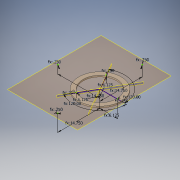
# Autodesk Inventor part: newCam08
Saved by Autodesk Inventor 2016 (Build 200138000, 138)
## iProperties
Created: 2015-07-25
Part Number: newCam08
Material: Generic
Document SubType Name: Modeling
Designer: steele
Density: 1 g/cm^3
Appearance: Default
Author: steele
Autodesk Inventor part; units mm, degrees
ref_plane "YZ Plane" through (0, 0, 0) normal (1, 0, 0) x (0, 1, 0)
ref_plane "XY Plane" through (0, 0, 0) normal (0, 0, 1) x (1, 0, 0)
sketch "Sketch1" plane through (0, 0, 0) normal (0, 1, 0) x (-1, 0, 0)
  circle A0 centre (0, 0) radius 149.225
  circle A1 centre (0, 0) radius 187.325
  dimension "insideCamDiam" = 298.45
  dimension "outsideCamDiam" = 374.65
  constraints: 2 centre point, 1 coincident
  measures "insideCamDiam" diameter of A0
  measures "outsideCamDiam" diameter of A1
extrude "Extrusion1" add sketch "Sketch1" against normal blind 12.7
sketch "Sketch yz neg" plane through (0, 0, 0) normal (1, 0, 0) x (0, 1, 0)
  circle A0 centre (0, -374.65) radius 3.175
  point P0 (0, 0)
  dimension "trackDiam" = 6.35
  dimension "yzNetOutsideCamTrackRadius" = 374.65
  constraints: 1 centre point
  measures "trackDiam" diameter of A0
  measures "yzNetOutsideCamTrackRadius" distance of point (0, 0) A0.centre
sketch "Sketch xy neg" plane through (0, 0, 0) normal (0, 0, 1) x (1, 0, 0)
  circle A0 centre (-374.65, 0) radius 3.175
  point P0 (0, 0)
  dimension "xyNegTrackDiam" = 6.35
  dimension "xyNegOutsideCamTrackRadius" = 374.65
  constraints: 1 centre point
  measures "xyNegTrackDiam" diameter of A0
  measures "xyNegOutsideCamTrackRadius" distance of point (0, 0) A0.centre
sketch "Sketch yz pos" plane through (0, 0, 0) normal (1, 0, 0) x (0, 1, 0)
  circle A0 centre (0, 374.65) radius 3.175
  point P0 (0, 0)
  dimension "yzOutsideCamTrackRadius" = 374.65
  dimension "yzPosTrackDiam" = 6.35
  constraints: 1 centre point
  measures "yzOutsideCamTrackRadius" distance of A0.centre point (0, 0)
  measures "yzPosTrackDiam" diameter of A0
sketch "Sketch xy pos for 1st cam position" plane through (0, 0, 0) normal (0, 0, 1) x (1, 0, 0)
  circle A0 centre (155.575, 0) radius 3.175
  point P0 (0, 0)
  dimension "xyPosInsideCamTrackRadius" = 155.575
  dimension "xyPosTrackDiam_Inner" = 6.35
  constraints: 1 centre point
  measures "xyPosInsideCamTrackRadius" distance of A0.centre point (0, 0)
  measures "xyPosTrackDiam_Inner" diameter of A0
sketch "Sketch for cam position" plane through (0, 0, 0) normal (0, 1, 0) x (-1, 0, 0)
  line L0 (0, 0) -> (94.0312, -162.8668)
  line L1 (0, 0) -> (-188.076, 0)
  line L2 (0, 0) -> (94.5746, 163.8079)
  dimension "d55" = 120
  dimension "d56" = 120
  constraints: 6 end point, 1 horizontal
  measures "d55" angle of L0 L1
  measures "d56" angle of L2 L1
ref_plane "Work Plane for 2nd cam position" through (0, 0, 0) normal (0.8660254, 0, -0.5) x (-0.5, 0, -0.8660254)
ref_plane "Work Plane for 3rd cam position" through (0, 0, 0) normal (-0.8660254, 0, -0.5) x (-0.5, 0, 0.8660254)
sketch "Sketch for 2nd cam position" plane through (0, 0, 0) normal (0.8660254, 0, -0.5) x (-0.5, 0, -0.8660254)
  circle A0 centre (155.575, 0) radius 3.175
  point P0 (0, 0)
  dimension "secondCamTrackRadius" = 155.575
  dimension "secondCamTrackDiam" = 6.35
  constraints: 1 centre point
  measures "secondCamTrackRadius" distance of A0.centre point (0, 0)
  measures "secondCamTrackDiam" diameter of A0
sketch "Sketch for 3rd cam position" plane through (0, 0, 0) normal (-0.8660254, 0, -0.5) x (-0.5, 0, 0.8660254)
  circle A0 centre (155.575, 0) radius 3.175
  point P0 (0, 0)
  dimension "thirdCamTrackDiam" = 6.35
  dimension "thirdCamTrackRadius" = 155.575
  constraints: 1 centre point
  measures "thirdCamTrackDiam" diameter of A0
  measures "thirdCamTrackRadius" distance of A0.centre point (0, 0)
equation "\"trackDiam\" = camTrackDiam"
equation "\"yzNetOutsideCamTrackRadius\" = outsideCamTrackRadius"
equation "\"xyNegTrackDiam\" = camTrackDiam"
equation "\"xyNegOutsideCamTrackRadius\" = outsideCamTrackRadius"
equation "\"yzOutsideCamTrackRadius\" = outsideCamTrackRadius"
equation "\"yzPosTrackDiam\" = camTrackDiam"
equation "\"xyPosInsideCamTrackRadius\" = insideCamTrackRadius"
equation "\"xyPosTrackDiam_Inner\" = camTrackDiam"
equation "\"d55\" = one_third_of_circle"
equation "\"d56\" = one_third_of_circle"
equation "\"secondCamTrackRadius\" = insideCamTrackRadius"
equation "\"secondCamTrackDiam\" = camTrackDiam"
equation "\"thirdCamTrackDiam\" = camTrackDiam"
equation "\"thirdCamTrackRadius\" = insideCamTrackRadius"
equation "\"frisbeeOuterDiamter\" = 279.4"
equation "\"frisbeeHopperOutsideDiam\" = 292.1"
equation "\"one_third_of_circle\" = 120deg"
equation "\"camTrackDiam\" = 6.35"
equation "\"outsideCamTrackRadius\" = 374.65"
equation "\"insideCamTrackRadius\" = 155.575"
body "Solid1"
